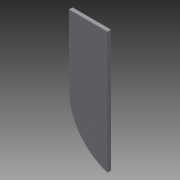
# Autodesk Inventor part: drzak_buzirka1
Saved by Autodesk Inventor 2015 (Build 190159000, 159)
## iProperties
Created: 2016-01-15
Part Number: drzak_buzirka1
Material: Generic
Document SubType Name: Modeling
Designer: Turboslimak
Density: 1 g/cm^3
Appearance: Default
Author: Turboslimak
Autodesk Inventor part; units mm, degrees
ref_plane "YZ Plane" through (0, 0, 0) normal (1, 0, 0) x (0, 1, 0)
ref_plane "XZ Plane" through (0, 0, 0) normal (0, 1, 0) x (-1, 0, 0)
ref_plane "XY Plane" through (0, 0, 0) normal (0, 0, 1) x (1, 0, 0)
sketch "Sketch1" plane through (0, 0, 0) normal (0, 1, 0) x (-1, 0, 0)
  line L0 (-11, -15) -> (-11, 15)
  line L1 (-11, 15) -> (11, 15)
  arc A0 (-11, -15) -> (11, 15) centre (-20.4545, 15) ccw
  line L2 (11, 15) -> (-11, 15)
  line L3 (-11, 15) -> (-11, 40)
  line L4 (-11, 40) -> (11, 40)
  line L5 (11, 40) -> (11, 15)
  line L6 (11, 40) -> (-11, 40)
  line L7 (-11, 40) -> (-11, 55)
  line L8 (-11, 55) -> (11, 55)
  line L9 (11, 55) -> (11, 40)
  circle A1 centre (0, 47.5) radius 0.1
  line L10 (-11, 15) -> (-3, 15)
  circle A2 centre (-3, 7) radius 0.1
  circle A3 centre (-3, -1) radius 0.1
  dimension "d0" = 22
  dimension "d1" = 30
  dimension "d2" = 25
  dimension "d3" = 15
  dimension "d4" = 0.2
  dimension "d5" = 8
  dimension "d8" = 0.2
  dimension "d10" = 0.2
  constraints: 22 end point, 4 centre point, 4 parallel, 2 horizontal, 2 perpendicular, 2 point on circle, 2 point on line
  measures "d0" distance of L0.end L1.end
  measures "d1" distance of L0.start L0.end
  measures "d2" distance of L2.end L3.end
  measures "d3" distance of L6.end L7.end
  measures "d4" diameter of A1
  measures "d5" distance of L2.end L10.end
  measures "d8" diameter of A2
  measures "d10" diameter of A3
extrude "Extrusion1" add sketch "Sketch1" along normal blind 2
body "Solid1"
